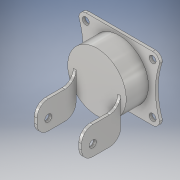
# Autodesk Inventor part: CastorBase
Saved by Autodesk Inventor 2018 (Build 220112000, 112)
## iProperties
Created: 2018-01-12
Part Number: CastorBase
Material: Stainless Steel
Document SubType Name: Modeling
Designer: Kyle
Density: 8 g/cm^3
Appearance: Aluminum - Polished
Author: Kyle
Autodesk Inventor part; units mm, degrees
ref_plane "YZ Plane" through (0, 0, 0) normal (1, 0, 0) x (0, 1, 0)
ref_plane "XZ Plane" through (0, 0, 0) normal (0, 1, 0) x (-1, 0, 0)
ref_plane "XY Plane" through (0, 0, 0) normal (0, 0, 1) x (1, 0, 0)
sketch "Sketch1" plane through (0, 0, 0) normal (0, 0, 1) x (1, 0, 0)
  arc A0 (33.655, 0) -> (30.48, 3.175) centre (30.48, 0) ccw
  arc A1 (0, 3.175) -> (-3.175, 0) centre (0, 0) ccw
  arc A2 (-3.175, -22.86) -> (0, -26.035) centre (0, -22.86) ccw
  arc A3 (30.48, -26.035) -> (33.655, -22.86) centre (30.48, -22.86) ccw
  line L0 (0, -26.035) -> (30.48, -26.035)
  line L1 (0, 3.175) -> (30.48, 3.175)
  arc A4 (-3.175, -22.86) -> (-3.175, 0) centre (-36.5125, -11.43) ccw
  arc A5 (33.655, 0) -> (33.655, -22.86) centre (66.9925, -11.43) ccw
  circle A6 centre (0, -22.86) radius 1.5875
  circle A7 centre (30.48, -22.86) radius 1.5875
  circle A8 centre (0, 0) radius 1.5875
  circle A9 centre (30.48, 0) radius 1.5875
  point P0 (31.75, -11.43)
  point P1 (-1.27, -11.43)
  dimension "d0" = 30.48
  dimension "d1" = 22.86
  dimension "d2" = 6.35
  dimension "d3" = 6.35
  dimension "d4" = 6.35
  dimension "d5" = 6.35
  dimension "d6" = 33.02
  dimension "d7" = 11.43
  dimension "d8" = 1.27
  dimension "d9" = 3.175
  dimension "d10" = 3.175
  dimension "d11" = 3.175
  dimension "d12" = 3.175
  constraints: 14 point on circle, 10 centre point, 9 coincident, 4 end point, 2 tangent, 1 horizontal, 1 parallel
  measures "d0" distance of point (0, 0) point (30.48, 0)
  measures "d1" distance of point (30.48, -22.86) point (30.48, 0)
  measures "d2" diameter of A0
  measures "d3" diameter of A1
  measures "d4" diameter of A2
  measures "d5" diameter of A3
  measures "d6" distance of point (31.75, -11.43) point (-1.27, -11.43)
  measures "d7" vertical distance of point (0, 0) point (-1.27, -11.43)
  measures "d8" horizontal distance of point (-1.27, -11.43) point (0, 0)
  measures "d9" diameter of A9
  measures "d10" diameter of A8
  measures "d11" diameter of A6
  measures "d12" diameter of A7
extrude "Extrusion1" add sketch "Sketch1" along normal blind 1.27
sketch "Sketch2" plane through (0, 0, 1.27) normal (0, 0, 1) x (1, 0, 0)
  circle A0 centre (15.24, -11.43) radius 13.335
  point P0 (0, 0)
  dimension "d15" = 26.67
  dimension "d16" = 15.24
  dimension "d17" = 11.43
  constraints: 1 centre point
  measures "d15" diameter of A0
  measures "d16" horizontal distance of point (0, 0) A0.centre
  measures "d17" vertical distance of point (0, 0) A0.centre
extrude "Extrusion2" add sketch "Sketch2" along normal blind 10.16
sketch "Sketch3" plane through (15.24, -11.43, 11.43) normal (0, 0, 1) x (1, 0, 0)
  line L0 (9.525, -5.08) -> (10.795, -5.08)
  line L1 (10.795, -5.08) -> (10.795, -17.78)
  line L2 (10.795, -17.78) -> (9.525, -17.78)
  line L3 (9.525, -17.78) -> (9.525, -5.08)
  line L4 (-10.795, -5.08) -> (-9.525, -5.08)
  line L5 (-9.525, -5.08) -> (-9.525, -17.78)
  line L6 (-9.525, -17.78) -> (-10.795, -17.78)
  line L7 (-10.795, -17.78) -> (-10.795, -5.08)
  circle A0 centre (0, 0) radius 13.335 projected
  point P0 (-15.24, 11.43)
  point P1 (-13.335, 0)
  dimension "d20" = 19.05
  dimension "d21" = 1.27
  dimension "d22" = 1.27
  dimension "d23" = 3.81
  dimension "d24" = 5.08
  dimension "d25" = 12.7
  constraints: 16 end point, 4 parallel, 2 collinear, 2 horizontal, 2 perpendicular, 1 horizontal alignment, 2 other
  measures "d20" distance between parallel lines of L5 L3
  measures "d21" distance of L0.start L0.end
  measures "d22" distance of L4.start L4.end
  measures "d23" distance from line of point (-13.335, 0) L5
  measures "d24" distance from line of point (0, 0) L0
  measures "d25" distance of L0.end L1.end
extrude "Extrusion3" add sketch "Sketch3" along normal blind 17.78 contours L0 L1 A0 L3 | A0 L1 L2 L3 | A0 L7 L4 L5 | L5 L6 L7 A0
sketch "Sketch4" plane through (26.035, -29.21, 11.43) normal (1, 0, 0) x (0, 0, -1)
  line L0 (0, 0) -> (-17.78, 0) projected
  line L1 (-17.78, 0) -> (-17.78, 12.7) projected
  circle A0 centre (-12.7, 5.08) radius 1.5875
  point P0 (11.43, 29.21)
  dimension "d28" = 5.08
  dimension "d29" = 5.08
  dimension "d30" = 3.175
  constraints: 1 centre point, 1 coincident
  measures "d28" distance from line of L0 point (-12.7, 5.08)
  measures "d29" distance from line of L1 point (-12.7, 5.08)
  measures "d30" diameter of A0
extrude "Extrusion4" cut sketch "Sketch4" against normal blind 50.8
fillet "Fillet1" radius 5.08 8 edges at (25.4, -29.21, 29.21) (5.08, -29.21, 29.21) (25.4, -16.51, 29.21) (5.08, -16.51, 29.21) (5.08, -16.51, 11.43) (25.4, -16.51, 11.43) (5.08, -29.21, 11.43) (25.4, -29.21, 11.43)
body "Solid1"
